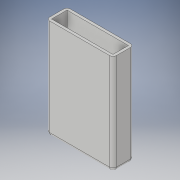
# Autodesk Inventor part: Mk2
Saved by Autodesk Inventor 2018 (Build 220112000, 112)
## iProperties
Created: 2018-01-10
Part Number: Mk2
Material: Generic
Document SubType Name: Modeling
Designer: mwood
Density: 1 g/cm^3
Appearance: Default
Author: mwood
Autodesk Inventor part; units mm, degrees
ref_plane "YZ Plane" through (0, 0, 0) normal (1, 0, 0) x (0, 1, 0)
ref_plane "XZ Plane" through (0, 0, 0) normal (0, 1, 0) x (-1, 0, 0)
ref_plane "XY Plane" through (0, 0, 0) normal (0, 0, 1) x (1, 0, 0)
sketch "Sketch1" plane through (0, 0, 0) normal (0, 0, 1) x (1, 0, 0)
  line L0 (0, 0) -> (63.754, 0)
  line L1 (63.754, 0) -> (63.754, 95.5802)
  line L2 (63.754, 95.5802) -> (0, 95.5802)
  line L3 (0, 95.5802) -> (0, 0)
  line L4 (4.6078, 104.8429) -> (58.4558, 104.8429)
  line L5 (58.4558, 104.8429) -> (58.4558, 3.2429)
  line L6 (58.4558, 3.2429) -> (4.6078, 3.2429)
  line L7 (4.6078, 3.2429) -> (4.6078, 104.8429)
  dimension "d0" = 63.754
  dimension "d1" = 95.5802
  dimension "d2" = 53.848
  dimension "d3" = 101.6
  constraints: 16 end point, 4 parallel, 2 perpendicular, 1 horizontal
  measures "d0" distance of L1.end L2.end
  measures "d1" distance of L0.end L1.end
  measures "d2" distance of L5.end L6.end
  measures "d3" distance of L4.end L5.end
extrude "Extrusion1" add sketch "Sketch1" along normal blind 19.812 contours L3 L2 L7 L6 L5 L1 L0 | L2 L5 L6 L7
shell "Shell1" thickness 2.54 removed faces 1 at (42.5027, 95.5802, 6.604)
fillet "Fillet1" radius 3.175 8 edges at (63.754, 47.7901, 19.812) (0, 47.7901, 19.812) (63.754, 47.7901, 0) (0, 47.7901, 0) (31.877, 0, 0) (63.754, 0, 9.906) (0, 0, 9.906) (31.877, 0, 19.812)
body "Solid1"
